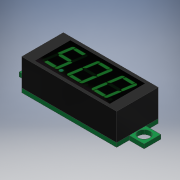
# Autodesk Inventor part: LED DC Digital Voltmeter 5V Display
Saved by Autodesk Inventor 2019 (Build 230136000, 136)
## iProperties
Created: 2018-10-18
Part Number: LED DC Digital Voltmeter 5V Display
Material: Allgemein
Document SubType Name: Modeling
Designer: KHG
Mass: 1.81968 g
Surface Area: 14.9296 cm^2
Volume: 1.81968 cm^3
Density: 1 g/cm^3
Appearance: Vorgabe
Catalog Web Link: https://www.amazon.de/gp/product/B076BGGT91/ref=oh_aui_detailpage_o00_s00?ie=UTF8&psc=1
Description: LED DC Digital Voltmeter 5V Display
Toleranz1: DIN ISO
Toleranz2: 2768-m
Artikelnummer: LX113655SFCIL1207
Kosten € pro Stück: 2,60
Kosten € Gesamt: 2,60
Author: KHG
Autodesk Inventor part; units mm, degrees
ref_plane "YZ Plane" through (0, 0, 0) normal (1, 0, 0) x (0, 1, 0)
ref_plane "XZ Plane" through (0, 0, 0) normal (0, 1, 0) x (-1, 0, 0)
ref_plane "XY Plane" through (0, 0, 0) normal (0, 0, 1) x (1, 0, 0)
sketch "Skizze1" plane through (0, 0, 0) normal (0, 0, 1) x (1, 0, 0)
  line L0 (-15.96, 0) -> (15.96, 0) construction
  line L1 (0, -7.0079) -> (0, 7.0013) construction
  line L2 (-11.4, 5) -> (11.4, 5)
  line L3 (11.4, 5) -> (11.4, -5)
  line L4 (11.4, -5) -> (-11.4, -5)
  line L5 (-11.4, -5) -> (-11.4, 5)
  point P0 (0, 0)
  dimension "d0" = 22.8
  dimension "d1" = 10
  constraints: 8 end point, 2 parallel, 1 horizontal, 1 perpendicular, 2 other
  measures "d0" distance of L2.start L2.end
  measures "d1" distance of L2.end L3.end
extrude "Extrusion1" add sketch "Skizze1" against normal blind 6.5
sketch "Skizze2" plane through (0, 0, -6.5) normal (0, 0, -1) x (-1, 0, 0)
  line L0 (-11.4, -5) -> (11.4, -5) construction
  line L1 (-11.4, 5) -> (-11.4, -5) construction
  line L2 (11.4, 5) -> (-11.4, 5) construction
  line L3 (11.4, -5) -> (11.4, 5) construction
  line L4 (21, 0) -> (-21, 0) construction
  line L5 (0, -7.0079) -> (0, 7.0013) construction
  line L6 (-11.4, -5) -> (11.4, -5)
  line L7 (11.4, 5) -> (-11.4, 5)
  line L8 (-11.4, -2) -> (-15, -2)
  line L9 (-15, -2) -> (-15, 2)
  line L10 (-15, 2) -> (-11.4, 2)
  line L11 (11.4, 2) -> (15, 2)
  line L12 (15, 2) -> (15, -2)
  line L13 (15, -2) -> (11.4, -2)
  circle A0 centre (-13, 0) radius 1.4
  circle A1 centre (13, 0) radius 1.15
  line L14 (-11.4, 5) -> (-11.4, 2)
  line L15 (-11.4, -2) -> (-11.4, -5)
  line L16 (11.4, -5) -> (11.4, -2)
  line L17 (11.4, 2) -> (11.4, 5)
  point P0 (0, 0)
  dimension "d4" = 4
  dimension "d6" = 30
  dimension "d7" = 2.8
  dimension "d8" = 2.3
  dimension "d9" = 26
  constraints: 24 end point, 7 parallel, 4 perpendicular, 4 point on line, 3 horizontal, 2 centre point, 2 collinear, 1 symmetric about line, 2 other
  measures "d4" distance of L8.end L9.end
  measures "d6" distance between parallel lines of L12 L9
  measures "d7" diameter of A0
  measures "d8" diameter of A1
  measures "d9" distance of A1.centre A0.centre
extrude "Extrusion2" add sketch "Skizze2" along normal blind 1 separate body
sketch "Skizze3" plane through (0, 0, 0) normal (0, 0, 1) x (1, 0, 0)
  line L0 (-8.9441, 4.2214) -> (8.9948, 4.2214) construction
  line L1 (8.9948, 4.2214) -> (8.9948, -4.2459) construction
  line L2 (8.9948, -4.2459) -> (-8.9441, -4.2459) construction
  line L3 (-8.9441, -4.2459) -> (-8.9441, 4.2214) construction
  point P0 (0, 0)
  constraints: 2 other
decal "Aufkleber1"
